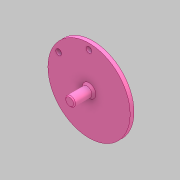
# Autodesk Inventor part: EncoderDisk
Saved by Autodesk Inventor 2018 (Build 220112000, 112)
## iProperties
Created: 2019-06-28
Part Number: EncoderDisk
Material: Generic
Document SubType Name: Modeling
Designer: mkivekas
Density: 1 g/cm^3
Appearance: Pink
Author: mkivekas
Autodesk Inventor part; units mm, degrees
ref_plane "YZ Plane" through (0, 0, 0) normal (1, 0, 0) x (0, 1, 0)
ref_plane "XZ Plane" through (0, 0, 0) normal (0, 1, 0) x (-1, 0, 0)
ref_plane "XY Plane" through (0, 0, 0) normal (0, 0, 1) x (1, 0, 0)
sketch "Sketch1" plane through (0, 0, 0) normal (0, 1, 0) x (-1, 0, 0)
  circle A0 centre (0, 0) radius 21.25
  circle A1 centre (0, 0) radius 18.25
  point P0 (0, 18.25)
  point P1 (15.676, 9.3448)
  dimension "d0" = 42.5
  dimension "d3" = 3
  dimension "d4" = 59.2
  constraints: 3 coincident, 2 centre point, 2 point on circle
  measures "d0" diameter of A0
  measures "d3" radial gap between concentric circles of A0 A1
extrude "Extrusion1" add sketch "Sketch1" along normal blind 2 contours A0 | A1
hole "Hole1" at (0, 0, 18.25) at (-15.676, 0, 9.3448) direction (0, 1, 0) diameter 3 depth 8 tip angle 118
sketch "Sketch2" plane through (0, 0, 0) normal (0, -1, 0) x (1, 0, 0)
  circle A0 centre (0, 0) radius 2.5
  dimension "d19" = 5
  constraints: 1 centre point, 1 coincident
  measures "d19" diameter of A0
extrude "Extrusion2" add sketch "Sketch2" along normal blind 10 and the other way blind 11
chamfer "Chamfer1" distance 1 angle 45 2 edges at (-2.5, 0, 0) (-2.5, 2, 0)
chamfer "Chamfer2" distance 0.5 angle 45 2 edges at (-2.5, 11, 0) (-2.5, -10, 0)
body "Solid1"
